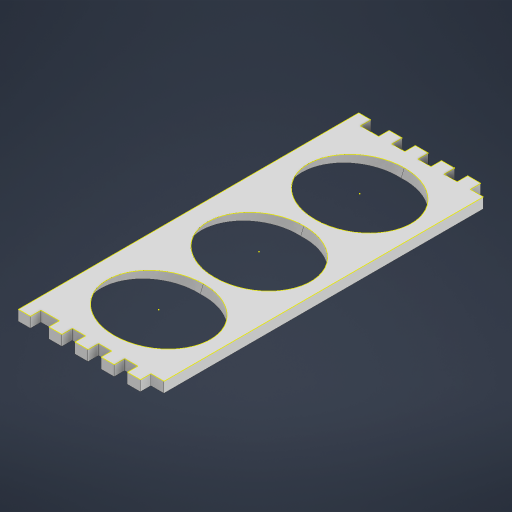
# Autodesk Inventor part: Angle Cover
Saved by Autodesk Inventor 2023 (Build 270158030, 158C)
## iProperties
Created: 2022-06-21
Part Number: Angle Cover
Material: Generic
Document SubType Name: Modeling
Designer: Simon
Density: 1 g/cm^3
Appearance: Default
Author: Simon
Autodesk Inventor part; units mm, degrees
ref_plane "YZ Plane" through (0, 0, 0) normal (1, 0, 0) x (0, 1, 0)
ref_plane "XZ Plane" through (0, 0, 0) normal (0, 1, 0) x (-1, 0, 0)
ref_plane "XY Plane" through (0, 0, 0) normal (0, 0, 1) x (1, 0, 0)
sketch "Sketch1" plane through (0, 0, 0) normal (0, 1, 0) x (-1, 0, 0)
  line L0 (-15, 0) -> (-15, 130)
  line L1 (-10, 0) -> (-10, 4)
  line L2 (-15, 4) -> (-10, 4)
  line L3 (-5, 0) -> (-10, 0)
  line L4 (-5, 0) -> (-5, 4)
  line L5 (-5, 4) -> (0, 4)
  line L6 (0, 0) -> (0, 4)
  line L7 (5, 0) -> (0, 0)
  line L8 (5, 0) -> (5, 4)
  line L9 (5, 4) -> (10, 4)
  line L10 (10, 0) -> (10, 4)
  line L11 (15, 0) -> (10, 0)
  line L12 (15, 0) -> (15, 4)
  line L13 (15, 4) -> (20, 4)
  line L14 (25, 0) -> (20, 0)
  line L15 (20, 0) -> (20, 4)
  line L16 (25, 0) -> (25, 4)
  line L17 (25, 4) -> (32, 4)
  line L18 (32, 0) -> (32, 4)
  line L19 (36.6188, 0) -> (32, 0)
  line L20 (36.6188, 0) -> (36.6188, 4)
  line L21 (36.6188, 4) -> (36.6188, 126)
  line L22 (36.6188, 126) -> (36.6188, 130)
  line L23 (32, 130) -> (36.6188, 130)
  line L24 (32, 126) -> (32, 130)
  line L25 (32, 126) -> (25, 126)
  line L26 (25, 126) -> (25, 130)
  line L27 (25, 130) -> (20, 130)
  line L28 (20, 126) -> (20, 130)
  line L29 (20, 126) -> (15, 126)
  line L30 (15, 126) -> (15, 130)
  line L31 (15, 130) -> (10, 130)
  line L32 (10, 126) -> (10, 130)
  line L33 (10, 126) -> (5, 126)
  line L34 (5, 126) -> (5, 130)
  line L35 (5, 130) -> (0, 130)
  line L36 (0, 126) -> (0, 130)
  line L37 (0, 126) -> (-5, 126)
  line L38 (-5, 126) -> (-5, 130)
  line L39 (-5, 130) -> (-10, 130)
  line L40 (-10, 126) -> (-10, 130)
  line L41 (-10, 126) -> (-15, 126)
  constraints: 84 end point
extrude "Extrusion1" add sketch "Sketch1" along normal blind 4
ref_plane "Work Plane1" through (15, 4, 130) normal (0.5, 0.8660254, 0) x (0, 0, -1)
sketch "Sketch3" plane through (15, 4, 130) normal (0.5, 0.8660254, 0) x (0, 0, -1)
  circle A0 centre (26.6791, -58.7868) radius 17.0835
  circle A1 centre (26.6813, 21.3732) radius 17.0835
  circle A2 centre (65.0579, 21.3722) radius 17.0835
  circle A3 centre (103.4345, 21.3711) radius 17.0835
  circle A4 centre (103.4323, -58.7889) radius 17.0835
  circle A5 centre (65.0557, -58.7878) radius 17.0835
  circle A6 centre (65.0568, -18.7078) radius 17.0835
  circle A7 centre (103.4334, -18.7089) radius 17.0835
  circle A8 centre (26.6802, -18.7068) radius 17.0835
  circle A9 centre (103.4313, -98.8689) radius 17.0835
  circle A10 centre (26.6781, -98.8668) radius 17.0835
  circle A11 centre (65.0547, -98.8678) radius 17.0835
  line L0 (8.1459, 47.2539) -> (3.022, 47.2539)
  line L1 (3.022, 47.2539) -> (3.0218, 40.2505)
  line L2 (3.0218, 40.2505) -> (-0.8586, 40.2505)
  line L3 (-0.8586, 40.2505) -> (-0.8586, 35.2505)
  line L4 (-0.8586, 35.2505) -> (3.0217, 35.2505)
  line L5 (3.0217, 35.2505) -> (3.0215, 30.2505)
  line L6 (3.0215, 30.2505) -> (-0.8586, 30.2505)
  line L7 (-0.8586, 30.2505) -> (-0.8586, 25.2505)
  line L8 (-0.8586, 25.2505) -> (3.0214, 25.2505)
  line L9 (3.0214, 25.2505) -> (3.0212, 20.2505)
  line L10 (3.0212, 20.2505) -> (-0.8586, 20.2505)
  line L11 (-0.8586, 20.2505) -> (-0.8586, 15.2505)
  line L12 (-0.8586, 15.2505) -> (3.0211, 15.2505)
  line L13 (3.0211, 15.2505) -> (3.021, 10.2505)
  line L14 (3.021, 10.2505) -> (-0.8586, 10.2505)
  line L15 (-0.8586, 10.2505) -> (-0.8586, 5.2505)
  line L16 (-0.8586, 5.2505) -> (3.0208, 5.2505)
  line L17 (3.0208, 5.2505) -> (3.0207, 0.2505)
  line L18 (3.0207, 0.2505) -> (-0.8586, 0.2505)
  line L19 (-0.8586, 0.2505) -> (-0.8586, -4.7495)
  line L20 (-0.8586, -4.7495) -> (3.0206, -4.7495)
  line L21 (3.0206, -4.7495) -> (3.0204, -9.7495)
  line L22 (3.0204, -9.7495) -> (-0.8586, -9.7495)
  line L23 (-0.8586, -9.7495) -> (-0.8586, -14.7495)
  line L24 (-0.8586, -14.7495) -> (3.0203, -14.7495)
  line L25 (3.0203, -14.7495) -> (3.0202, -19.7495)
  line L26 (3.0202, -19.7495) -> (-0.8586, -19.7495)
  line L27 (-0.8586, -19.7495) -> (-0.8586, -24.7495)
  line L28 (-0.8586, -24.7495) -> (3.02, -24.7495)
  line L29 (3.02, -24.7495) -> (3.0199, -29.7495)
  line L30 (3.0199, -29.7495) -> (-0.8586, -29.7495)
  line L31 (-0.8586, -29.7495) -> (-0.8586, -34.7495)
  line L32 (-0.8586, -34.7495) -> (3.0197, -34.7495)
  line L33 (3.0197, -34.7495) -> (3.0196, -39.7495)
  line L34 (3.0196, -39.7495) -> (-0.8586, -39.7495)
  line L35 (-0.8586, -39.7495) -> (-0.8586, -44.7495)
  line L36 (-0.8586, -44.7495) -> (3.0195, -44.7495)
  line L37 (3.0195, -44.7495) -> (3.0193, -49.7495)
  line L38 (3.0193, -49.7495) -> (-0.8586, -49.7495)
  line L39 (-0.8586, -49.7495) -> (-0.8586, -54.7495)
  line L40 (-0.8586, -54.7495) -> (3.0192, -54.7495)
  line L41 (3.0192, -54.7495) -> (3.0191, -59.7495)
  line L42 (3.0191, -59.7495) -> (-0.8586, -59.7495)
  line L43 (-0.8586, -59.7495) -> (-0.8586, -64.7495)
  line L44 (-0.8586, -64.7495) -> (3.0189, -64.7495)
  line L45 (3.0189, -64.7495) -> (3.0188, -69.7495)
  line L46 (3.0188, -69.7495) -> (-0.8586, -69.7495)
  line L47 (-0.8586, -69.7495) -> (-0.8586, -74.7495)
  line L48 (-0.8586, -74.7495) -> (3.0187, -74.7495)
  line L49 (3.0187, -74.7495) -> (3.0185, -79.7495)
  line L50 (3.0185, -79.7495) -> (-0.8586, -79.7495)
  line L51 (-0.8586, -79.7495) -> (-0.8586, -84.7495)
  line L52 (-0.8586, -84.7495) -> (3.0184, -84.7495)
  line L53 (3.0184, -84.7495) -> (3.0182, -89.7495)
  line L54 (3.0182, -89.7495) -> (-0.8586, -89.7495)
  line L55 (-0.8586, -89.7495) -> (-0.8586, -94.7495)
  line L56 (-0.8586, -94.7495) -> (3.0181, -94.7495)
  line L57 (3.0181, -94.7495) -> (3.018, -99.7495)
  line L58 (3.018, -99.7495) -> (-0.8586, -99.7495)
  line L59 (-0.8586, -99.7495) -> (-0.8586, -104.7495)
  line L60 (-0.8586, -104.7495) -> (3.0178, -104.7495)
  line L61 (3.0178, -104.7495) -> (3.0177, -109.7495)
  line L62 (3.0177, -109.7495) -> (-0.8586, -109.7495)
  line L63 (-0.8586, -109.7495) -> (-0.8586, -114.7495)
  line L64 (-0.8586, -114.7495) -> (3.0176, -114.7495)
  line L65 (3.0176, -114.7495) -> (3.0174, -119.7495)
  line L66 (3.0174, -119.7495) -> (-0.8586, -119.7495)
  line L67 (-0.8586, -119.7495) -> (-0.8586, -124.7495)
  line L68 (-0.8586, -124.7495) -> (7.1414, -124.7495)
  line L69 (7.1414, -124.7495) -> (7.1414, -120.9103)
  line L70 (7.1414, -120.9103) -> (12.1414, -120.9104)
  line L71 (12.1414, -120.9104) -> (12.1414, -124.7495)
  line L72 (12.1414, -124.7495) -> (17.1414, -124.7495)
  line L73 (17.1414, -124.7495) -> (17.1414, -120.9105)
  line L74 (17.1414, -120.9105) -> (22.1414, -120.9107)
  line L75 (22.1414, -120.9107) -> (22.1414, -124.7495)
  line L76 (22.1414, -124.7495) -> (27.1414, -124.7495)
  line L77 (27.1414, -124.7495) -> (27.1414, -120.9108)
  line L78 (27.1414, -120.9108) -> (32.1414, -120.9109)
  line L79 (32.1414, -120.9109) -> (32.1414, -124.7495)
  line L80 (32.1414, -124.7495) -> (37.1414, -124.7495)
  line L81 (37.1414, -124.7495) -> (37.1414, -120.9111)
  line L82 (37.1414, -120.9111) -> (42.1414, -120.9112)
  line L83 (42.1414, -120.9112) -> (42.1414, -124.7495)
  line L84 (42.1414, -124.7495) -> (47.1414, -124.7495)
  line L85 (47.1414, -124.7495) -> (47.1414, -120.9113)
  line L86 (47.1414, -120.9113) -> (52.1414, -120.9115)
  line L87 (52.1414, -120.9115) -> (52.1414, -124.7495)
  line L88 (52.1414, -124.7495) -> (57.1414, -124.7495)
  line L89 (57.1414, -124.7495) -> (57.1414, -120.9116)
  line L90 (57.1414, -120.9116) -> (62.1414, -120.9118)
  line L91 (62.1414, -120.9118) -> (62.1414, -124.7495)
  line L92 (62.1414, -124.7495) -> (67.1414, -124.7495)
  line L93 (67.1414, -124.7495) -> (67.1414, -120.9119)
  line L94 (67.1414, -120.9119) -> (72.1414, -120.912)
  line L95 (72.1414, -120.912) -> (72.1414, -124.7495)
  line L96 (72.1414, -124.7495) -> (77.1414, -124.7495)
  line L97 (77.1414, -124.7495) -> (77.1414, -120.9122)
  line L98 (77.1414, -120.9122) -> (82.1414, -120.9123)
  line L99 (82.1414, -120.9123) -> (82.1414, -124.7495)
  line L100 (82.1414, -124.7495) -> (87.1414, -124.7495)
  line L101 (87.1414, -124.7495) -> (87.1414, -120.9124)
  line L102 (87.1414, -120.9124) -> (92.1414, -120.9126)
  line L103 (92.1414, -120.9126) -> (92.1414, -124.7495)
  line L104 (92.1414, -124.7495) -> (97.1414, -124.7495)
  line L105 (97.1414, -124.7495) -> (97.1414, -120.9127)
  line L106 (97.1414, -120.9127) -> (102.1414, -120.9128)
  line L107 (102.1414, -120.9128) -> (102.1414, -124.7495)
  line L108 (102.1414, -124.7495) -> (107.1414, -124.7495)
  line L109 (107.1414, -124.7495) -> (107.1414, -120.913)
  line L110 (107.1414, -120.913) -> (112.1414, -120.9131)
  line L111 (112.1414, -120.9131) -> (112.1414, -124.7495)
  line L112 (112.1414, -124.7495) -> (117.1414, -124.7495)
  line L113 (117.1414, -124.7495) -> (117.1414, -120.9133)
  line L114 (117.1414, -120.9133) -> (122.1414, -120.9134)
  line L115 (122.1414, -120.9134) -> (122.1414, -124.7495)
  line L116 (122.1414, -124.7495) -> (127.2653, -124.7495)
  line L117 (127.2653, -124.7495) -> (127.2655, -117.7494)
  line L118 (127.2655, -117.7494) -> (131.1459, -117.7494)
  line L119 (131.1459, -117.7494) -> (131.1459, -112.7494)
  line L120 (131.1459, -112.7494) -> (127.2656, -112.7494)
  line L121 (127.2656, -112.7494) -> (127.2658, -107.7494)
  line L122 (127.2658, -107.7494) -> (131.1459, -107.7494)
  line L123 (131.1459, -107.7494) -> (131.1459, -102.7494)
  line L124 (131.1459, -102.7494) -> (127.2659, -102.7494)
  line L125 (127.2659, -102.7494) -> (127.266, -97.7494)
  line L126 (127.266, -97.7494) -> (131.1459, -97.7494)
  line L127 (131.1459, -97.7494) -> (131.1459, -92.7494)
  line L128 (131.1459, -92.7494) -> (127.2662, -92.7494)
  line L129 (127.2662, -92.7494) -> (127.2663, -87.7494)
  line L130 (127.2663, -87.7494) -> (131.1459, -87.7494)
  line L131 (131.1459, -87.7494) -> (131.1459, -82.7494)
  line L132 (131.1459, -82.7494) -> (127.2664, -82.7494)
  line L133 (127.2664, -82.7494) -> (127.2666, -77.7494)
  line L134 (127.2666, -77.7494) -> (131.1459, -77.7494)
  line L135 (131.1459, -77.7494) -> (131.1459, -72.7494)
  line L136 (131.1459, -72.7494) -> (127.2667, -72.7494)
  line L137 (127.2667, -72.7494) -> (127.2668, -67.7494)
  line L138 (127.2668, -67.7494) -> (131.1459, -67.7494)
  line L139 (131.1459, -67.7494) -> (131.1459, -62.7494)
  line L140 (131.1459, -62.7494) -> (127.267, -62.7494)
  line L141 (127.267, -62.7494) -> (127.2671, -57.7494)
  line L142 (127.2671, -57.7494) -> (131.1459, -57.7494)
  line L143 (131.1459, -57.7494) -> (131.1459, -52.7494)
  line L144 (131.1459, -52.7494) -> (127.2673, -52.7494)
  line L145 (127.2673, -52.7494) -> (127.2674, -47.7494)
  line L146 (127.2674, -47.7494) -> (131.1459, -47.7494)
  line L147 (131.1459, -47.7494) -> (131.1459, -42.7494)
  line L148 (131.1459, -42.7494) -> (127.2675, -42.7494)
  line L149 (127.2675, -42.7494) -> (127.2677, -37.7494)
  line L150 (127.2677, -37.7494) -> (131.1459, -37.7494)
  line L151 (131.1459, -37.7494) -> (131.1459, -32.7494)
  line L152 (131.1459, -32.7494) -> (127.2678, -32.7494)
  line L153 (127.2678, -32.7494) -> (127.2679, -27.7494)
  line L154 (127.2679, -27.7494) -> (131.1459, -27.7494)
  line L155 (131.1459, -27.7494) -> (131.1459, -22.7494)
  line L156 (131.1459, -22.7494) -> (127.2681, -22.7494)
  line L157 (127.2681, -22.7494) -> (127.2682, -17.7494)
  line L158 (127.2682, -17.7494) -> (131.1459, -17.7494)
  line L159 (131.1459, -17.7494) -> (131.1459, -12.7494)
  line L160 (131.1459, -12.7494) -> (127.2683, -12.7494)
  line L161 (127.2683, -12.7494) -> (127.2685, -7.7494)
  line L162 (127.2685, -7.7494) -> (131.1459, -7.7494)
  line L163 (131.1459, -7.7494) -> (131.1459, -2.7494)
  line L164 (131.1459, -2.7494) -> (127.2686, -2.7494)
  line L165 (127.2686, -2.7494) -> (127.2688, 2.2506)
  line L166 (127.2688, 2.2506) -> (131.1459, 2.2506)
  line L167 (131.1459, 2.2506) -> (131.1459, 7.2506)
  line L168 (131.1459, 7.2506) -> (127.2689, 7.2506)
  line L169 (127.2689, 7.2506) -> (127.269, 12.2506)
  line L170 (127.269, 12.2506) -> (131.1459, 12.2506)
  line L171 (131.1459, 12.2506) -> (131.1459, 17.2506)
  line L172 (131.1459, 17.2506) -> (127.2692, 17.2506)
  line L173 (127.2692, 17.2506) -> (127.2693, 22.2506)
  line L174 (127.2693, 22.2506) -> (131.1459, 22.2506)
  line L175 (131.1459, 22.2506) -> (131.1459, 27.2506)
  line L176 (131.1459, 27.2506) -> (127.2694, 27.2506)
  line L177 (127.2694, 27.2506) -> (127.2696, 32.2506)
  line L178 (127.2696, 32.2506) -> (131.1459, 32.2506)
  line L179 (131.1459, 32.2506) -> (131.1459, 37.2506)
  line L180 (131.1459, 37.2506) -> (127.2697, 37.2506)
  line L181 (127.2697, 37.2506) -> (127.2698, 42.2506)
  line L182 (127.2698, 42.2506) -> (131.1459, 42.2506)
  line L183 (131.1459, 42.2506) -> (131.1459, 47.2506)
  line L184 (131.1459, 47.2506) -> (123.1459, 47.2506)
  line L185 (123.1459, 47.2506) -> (123.1459, 43.4146)
  line L186 (123.1459, 43.4146) -> (118.1459, 43.4147)
  line L187 (118.1459, 43.4147) -> (118.1459, 47.2509)
  line L188 (118.1459, 47.2509) -> (113.1459, 47.2509)
  line L189 (113.1459, 47.2509) -> (113.1459, 43.4149)
  line L190 (113.1459, 43.4149) -> (108.1459, 43.415)
  line L191 (108.1459, 43.415) -> (108.1459, 47.2511)
  line L192 (108.1459, 47.2511) -> (103.1459, 47.2511)
  line L193 (103.1459, 47.2511) -> (103.1459, 43.4151)
  line L194 (103.1459, 43.4151) -> (98.1459, 43.4153)
  line L195 (98.1459, 43.4153) -> (98.1459, 47.2514)
  line L196 (98.1459, 47.2514) -> (93.1459, 47.2514)
  line L197 (93.1459, 47.2514) -> (93.1459, 43.4154)
  line L198 (93.1459, 43.4154) -> (88.1459, 43.4155)
  line L199 (88.1459, 43.4155) -> (88.1459, 47.2517)
  line L200 (88.1459, 47.2517) -> (83.1459, 47.2517)
  line L201 (83.1459, 47.2517) -> (83.1459, 43.4157)
  line L202 (83.1459, 43.4157) -> (78.1459, 43.4158)
  line L203 (78.1459, 43.4158) -> (78.1459, 47.2519)
  line L204 (78.1459, 47.2519) -> (73.1459, 47.2519)
  line L205 (73.1459, 47.2519) -> (73.1459, 43.4159)
  line L206 (73.1459, 43.4159) -> (68.1459, 43.4161)
  line L207 (68.1459, 43.4161) -> (68.1459, 47.2522)
  line L208 (68.1459, 47.2522) -> (63.1459, 47.2522)
  line L209 (63.1459, 47.2522) -> (63.1459, 43.4162)
  line L210 (63.1459, 43.4162) -> (58.1459, 43.4164)
  line L211 (58.1459, 43.4164) -> (58.1459, 47.2525)
  line L212 (58.1459, 47.2525) -> (53.1459, 47.2525)
  line L213 (53.1459, 47.2525) -> (53.1459, 43.4165)
  line L214 (53.1459, 43.4165) -> (48.1459, 43.4166)
  line L215 (48.1459, 43.4166) -> (48.1459, 47.2528)
  line L216 (48.1459, 47.2528) -> (43.1459, 47.2528)
  line L217 (43.1459, 47.2528) -> (43.1459, 43.4168)
  line L218 (43.1459, 43.4168) -> (38.1459, 43.4169)
  line L219 (38.1459, 43.4169) -> (38.1459, 47.253)
  line L220 (38.1459, 47.253) -> (33.1459, 47.253)
  line L221 (33.1459, 47.253) -> (33.1459, 43.417)
  line L222 (33.1459, 43.417) -> (28.1459, 43.4172)
  line L223 (28.1459, 43.4172) -> (28.1459, 47.2533)
  line L224 (28.1459, 47.2533) -> (23.1459, 47.2533)
  line L225 (23.1459, 47.2533) -> (23.1459, 43.4173)
  line L226 (23.1459, 43.4173) -> (18.1459, 43.4174)
  line L227 (18.1459, 43.4174) -> (18.1459, 47.2536)
  line L228 (18.1459, 47.2536) -> (13.1459, 47.2536)
  line L229 (13.1459, 47.2536) -> (13.1459, 43.4176)
  line L230 (13.1459, 43.4176) -> (8.1459, 43.4177)
  line L231 (8.1459, 43.4177) -> (8.1459, 47.2539)
  point P0 (130, 10.9904)
  point P1 (65.057, -18.7478)
  dimension "d3" = 132.0045
  dimension "d4" = 172.0034
  dimension "d5" = 7.0034
  dimension "d6" = 3.8804
  dimension "d7" = 47.0034
  dimension "d8" = 125
  dimension "d9" = 5
  dimension "d10" = 7.0001
  dimension "d11" = 8
  constraints: 464 end point, 12 centre point
  measures "d3" distance between parallel lines of L183 L3
  measures "d4" distance between parallel lines of L0 L68
  measures "d5" distance of L0.end L1.end
  measures "d6" distance of L1.end L2.end
  measures "d7" distance between parallel lines of L0 L18
  measures "d8" distance between parallel lines of L68 L18
  measures "d9" distance of L66.end L67.end
  measures "d10" distance of L116.end L117.end
  measures "d11" distance of L183.end L184.end
extrude "Extrusion2" cut sketch "Sketch3" against normal blind 31.75 contours A1 | A2 | A3
sketch "Sketch4" plane through (0, 4, 0) normal (0, 1, 0) x (1, 0, 0)
  ellipse E0 centre (-9.6797, -103.3187) end of major axis (10.0467, -103.3187) minor radius 17.0835 projected
  ellipse E1 centre (-9.6785, -64.9421) end of major axis (10.0479, -64.9421) minor radius 17.0835 projected
  ellipse E2 centre (-9.6772, -26.5655) end of major axis (10.0491, -26.5655) minor radius 17.0835 projected
  point P0 (0, 0)
extrude "Extrusion3" cut sketch "Sketch4" against normal blind 31.75
sketch "Sketch5" plane through (0, 4, 0) normal (0, 1, 0) x (1, 0, 0)
  ellipse E0 centre (-9.6772, -26.5655) end of major axis (10.0491, -26.5655) minor radius 17.0835 (-9.6772, -9.482) -> (-9.6772, -43.649) ccw projected
  ellipse E1 centre (-9.6772, -26.5655) end of major axis (10.0491, -26.5655) minor radius 17.0835 (-9.6772, -43.649) -> (-9.6772, -9.482) ccw projected
  ellipse E2 centre (-9.6785, -64.9421) end of major axis (10.0479, -64.9421) minor radius 17.0835 (-9.6785, -47.8586) -> (-9.6785, -82.0256) ccw projected
  ellipse E3 centre (-9.6785, -64.9421) end of major axis (10.0479, -64.9421) minor radius 17.0835 (-9.6785, -82.0256) -> (-9.6785, -47.8586) ccw projected
  ellipse E4 centre (-9.6797, -103.3187) end of major axis (10.0467, -103.3187) minor radius 17.0835 (-9.6797, -86.2352) -> (-9.6797, -120.4022) ccw projected
  ellipse E5 centre (-9.6797, -103.3187) end of major axis (10.0467, -103.3187) minor radius 17.0835 (-9.6797, -120.4022) -> (-9.6797, -86.2352) ccw projected
  line L0 (10, 0) -> (5, 0) projected
  line L1 (5, 0) -> (5, -4) projected
  line L2 (5, -4) -> (0, -4) projected
  line L3 (0, -4) -> (0, 0) projected
  line L4 (0, 0) -> (-5, 0) projected
  line L5 (-5, 0) -> (-5, -4) projected
  line L6 (-5, -4) -> (-10, -4) projected
  line L7 (-10, -4) -> (-10, 0) projected
  line L8 (-10, 0) -> (-15, 0) projected
  line L9 (-15, 0) -> (-15, -4) projected
  line L10 (-15, -4) -> (-20, -4) projected
  line L11 (-20, -4) -> (-20, 0) projected
  line L12 (-20, 0) -> (-25, 0) projected
  line L13 (-25, 0) -> (-25, -4) projected
  line L14 (-25, -4) -> (-32, -4) projected
  line L15 (-32, -4) -> (-32, 0) projected
  line L16 (-32, 0) -> (-36.6188, 0) projected
  line L17 (-36.6188, 0) -> (-36.6188, -130) projected
  line L18 (-36.6188, -130) -> (-32, -130) projected
  line L19 (-32, -130) -> (-32, -126) projected
  line L20 (-32, -126) -> (-25, -126) projected
  line L21 (-25, -126) -> (-25, -130) projected
  line L22 (-25, -130) -> (-20, -130) projected
  line L23 (-20, -130) -> (-20, -126) projected
  line L24 (-20, -126) -> (-15, -126) projected
  line L25 (-15, -126) -> (-15, -130) projected
  line L26 (-15, -130) -> (-10, -130) projected
  line L27 (-10, -130) -> (-10, -126) projected
  line L28 (-10, -126) -> (-5, -126) projected
  line L29 (-5, -126) -> (-5, -130) projected
  line L30 (-5, -130) -> (0, -130) projected
  line L31 (0, -130) -> (0, -126) projected
  line L32 (0, -126) -> (5, -126) projected
  line L33 (5, -126) -> (5, -130) projected
  line L34 (5, -130) -> (10, -130) projected
  line L35 (10, -130) -> (10, -126) projected
  line L36 (10, -126) -> (15, -126) projected
  line L37 (15, -126) -> (15, -4) projected
  line L38 (15, -4) -> (10, -4) projected
  line L39 (10, -4) -> (10, 0) projected
  constraints: 6 other
body "Solid1"
